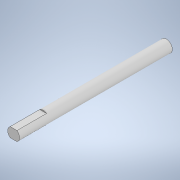
# Autodesk Inventor part: oś napędowa 12mm
Saved by Autodesk Inventor 2021 (Build 250183000, 183)
## iProperties
Created: 2021-06-25
Part Number: oś napędowa 12mm
Material: Generic
Document SubType Name: Modeling
Designer: Łukasz
Density: 1 g/cm^3
Appearance: Default
Author: Łukasz
Autodesk Inventor part; units mm, degrees
ref_plane "YZ Plane" through (0, 0, 0) normal (1, 0, 0) x (0, 1, 0)
ref_plane "XZ Plane" through (0, 0, 0) normal (0, 1, 0) x (-1, 0, 0)
ref_plane "XY Plane" through (0, 0, 0) normal (0, 0, 1) x (1, 0, 0)
sketch "Sketch1" plane through (0, 0, 0) normal (0, 0, 1) x (1, 0, 0)
  circle A0 centre (0, 0) radius 6
  dimension "d0" = 12
  constraints: 1 centre point, 1 coincident
  measures "d0" diameter of A0
extrude "Extrusion1" add sketch "Sketch1" along normal blind 155
sketch "Sketch2" plane through (0, 0, 155) normal (0, 0, 1) x (1, 0, 0)
  arc A0 (-3.4627, 4.9) -> (-3.4627, -4.9) centre (0, 0) ccw
  line L0 (-3.4627, 4.9) -> (3.4627, 4.9)
  arc A1 (3.4627, -4.9) -> (3.4627, 4.9) centre (0, 0) ccw
  line L1 (3.4627, -4.9) -> (-3.4627, -4.9)
  line L2 (-4.1729, 7.0025) -> (4.0866, 7.0025)
  line L3 (4.0866, 7.0025) -> (4.0866, 4.9)
  line L4 (4.0866, 4.9) -> (-4.1729, 4.9)
  line L5 (-4.1729, 4.9) -> (-4.1729, 7.0025)
  line L6 (-3.9468, -4.9) -> (4.2356, -4.9)
  line L7 (4.2356, -4.9) -> (4.2356, -6.7965)
  line L8 (4.2356, -6.7965) -> (-3.9468, -6.7965)
  line L9 (-3.9468, -6.7965) -> (-3.9468, -4.9)
  point P0 (-3.4627, 4.9)
  point P1 (3.4627, -4.9)
  point P2 (-3.4627, -4.9)
  constraints: 20 end point, 4 parallel, 4 point on circle, 2 centre point, 2 horizontal, 2 perpendicular
extrude "Extrusion2" cut sketch "Sketch2" against normal blind 30 contours L4 L5 L2 L3 L0 | L1 L6 L7 L8 L9
body "Solid1"
